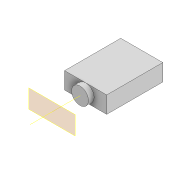
# Autodesk Inventor part: HandY
Saved by Autodesk Inventor 2021 (Build 250183000, 183)
## iProperties
Created: 2020-12-19
Part Number: HandY
Material: 一般
Document SubType Name: Modeling
Designer: Tazaki
Density: 2.15454 g/cm^3
Appearance: 既定
Mass: 500 g
Surface Area: 264.425 cm^2
Volume: 232.069 cm^3
Author: Tazaki
Autodesk Inventor part; units mm, degrees
ref_plane "YZ Plane" through (0, 0, 0) normal (1, 0, 0) x (0, 1, 0)
ref_plane "XZ Plane" through (0, 0, 0) normal (0, 1, 0) x (-1, 0, 0)
sketch "スケッチ2" plane through (0, 0, 0) normal (0, 0, 1) x (1, 0, 0)
  circle A0 centre (0, 0) radius 15
  dimension "d2" = 30
  constraints: 1 centre point, 1 coincident
  measures "d2" diameter of A0
extrude "押し出し1" add sketch "スケッチ2" against normal blind 60
sketch "スケッチ3" plane through (0, 0, -60) normal (0, 0, -1) x (-1, 0, 0)
  line L0 (37.5, 15) -> (-37.5, 15)
  line L1 (-37.5, 15) -> (-37.5, -15)
  line L2 (-37.5, -15) -> (37.5, -15)
  line L3 (37.5, -15) -> (37.5, 15)
  point P0 (0, 0)
  point P1 (0, 15)
  point P2 (37.5, 0)
  dimension "d5" = 30
  dimension "d6" = 75
  constraints: 8 end point, 2 midpoint, 2 parallel, 1 horizontal, 1 horizontal alignment, 1 perpendicular, 1 vertical alignment
  measures "d5" distance of L2.end L0.start
  measures "d6" distance of L0.start L0.end
extrude "押し出し2" add sketch "スケッチ3" along normal blind 100
sketch "スケッチ4" plane through (0, 0, 0) normal (0, 1, 0) x (-1, 0, 0)
  line L0 (63.5061, 71.4951) -> (-75.4219, 71.4951)
  line L1 (-75.4219, 71.4951) -> (-75.4219, -50)
  line L2 (-75.4219, -50) -> (63.5061, -50)
  line L3 (63.5061, -50) -> (63.5061, 71.4951)
  line L4 (-103.2075, 0) -> (91.2917, 0) projected
  point P0 (0, 0)
  dimension "d9" = 50
  constraints: 8 end point, 2 parallel, 1 horizontal, 1 perpendicular
  measures "d9" distance between parallel lines of L2 L4
extrude "押し出し3" cut sketch "スケッチ4" against normal mid plane 100
